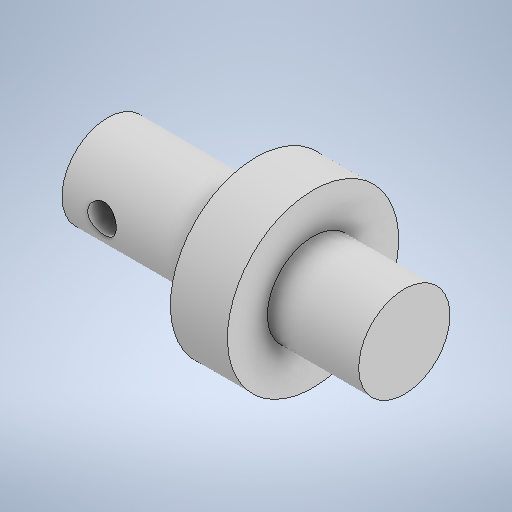
# Autodesk Inventor part: Pieza 10
Saved by Autodesk Inventor 2025.3 (Build 293356030, 356C)
## iProperties
Created: 2025-08-24
Part Number: Pieza 10
Material: Generic
Document SubType Name: Modeling
Designer: PC
Density: 1 g/cm^3
Appearance: Default
Author: PC
Autodesk Inventor part; units mm, degrees
ref_plane "YZ Plane" through (0, 0, 0) normal (1, 0, 0) x (0, 1, 0)
ref_plane "XZ Plane" through (0, 0, 0) normal (0, 1, 0) x (-1, 0, 0)
ref_plane "XY Plane" through (0, 0, 0) normal (0, 0, 1) x (1, 0, 0)
sketch "Sketch1" plane through (0, 0, 0) normal (0, 0, 1) x (1, 0, 0)
  line L0 (-8, 7.5) -> (-13, 7.5)
  line L1 (-13, 7.5) -> (-13, 4)
  line L2 (-13, 4) -> (-26, 4)
  line L3 (-26, 4) -> (-26, 0)
  line L4 (-26, 0) -> (0, 0)
  line L5 (0, 0) -> (0, 4)
  line L6 (-8, 7.5) -> (-8, 4)
  line L7 (-8, 4) -> (0, 4)
  circle A0 centre (-22.5, 0) radius 1.25
  dimension "d2" = 4
  dimension "d3" = 4
  dimension "d4" = 8
  dimension "d5" = 5
  dimension "d6" = 13
  dimension "d7" = 7.5
  dimension "d8" = 2.5
  dimension "d9" = 3.5
  constraints: 16 end point, 3 perpendicular, 2 horizontal, 2 vertical, 1 centre point, 1 point on line
  measures "d2" distance of L4.end L5.end
  measures "d3" distance of L2.end L3.end
  measures "d4" distance of L6.end L5.end
  measures "d5" distance of L0.start L0.end
  measures "d6" distance of L1.end L2.end
  measures "d7" distance between parallel lines of L0 L4
  measures "d8" diameter of A0
  measures "d9" distance of A0.centre L3.end
revolve "Revolution1" add sketch "Sketch1" angle 360 about axis through (-26, 0, 0) along (1, 0, 0) picked at (-22.1881, 0.2763) contours L6 L7 L5 L4 A0 L3 L2 L1 L0 | L4 A0
extrude "Extrusion1" cut sketch "Sketch1" along normal mid plane 100 contours A0 L4 | L4 A0
body "Solid1"
